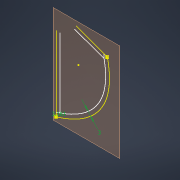
# Autodesk Inventor part: clamsheel sheet surface
Saved by Autodesk Inventor 2021 (Build 250183000, 183)
## iProperties
Created: 2021-02-13
Part Number: clamsheel sheet surface
Material: ABS Plastic
Document SubType Name: Modeling
Designer: vikki
Mass: 19.433 g
Surface Area: 131.842 cm^2
Volume: 18.333 cm^3
Density: 1.06 g/cm^3
Appearance: Brass - Satin
Author: vikki
Autodesk Inventor part; units mm, degrees
ref_plane "YZ Plane" through (0, 0, 0) normal (1, 0, 0) x (0, 1, 0)
ref_plane "XZ Plane" through (0, 0, 0) normal (0, 1, 0) x (-1, 0, 0)
ref_plane "XY Plane" through (0, 0, 0) normal (0, 0, 1) x (1, 0, 0)
ref_plane "Work Plane1" through (0, 0, 0) normal (0, 0, 1) x (1, 0, 0)
sketch "Sketch1" plane through (0, 0, 0) normal (0, 0, 1) x (1, 0, 0)
  spline S0 degree 3 poles (-17.5035, -43.75) (9.5564, -35.6427) (30.0035, -17.8707) (22.4965, 16.6912) knots 1 1 1 1 2 2 2 2 projected
  line L0 (22.4965, 16.6912) -> (-1.9986, 25.6067) projected
  line L1 (-17.5035, 14.75) -> (-17.5035, -43.75) projected
  line L2 (-3.0246, 22.7876) -> (19.8959, 14.4452)
  line L3 (-14.5035, -39.6343) -> (-14.5035, 14.75)
  line L4 (19.8959, 14.4452) -> (19.8959, 17.6377)
  line L5 (-14.5035, -39.6343) -> (-17.5035, -40.6309)
  spline S1 degree 5 poles (19.896, 14.4452) (20.6656, 10.4799) (21.1568, 6.4613) (21.3154, 2.402) (20.7956, -5.2165) (18.5576, -12.5026) (17.0978, -15.7703) (13.3907, -21.8782) (8.4101, -27.002) (5.6606, -29.2971) (0.173, -33.1415) (-5.7852, -36.2005) (-8.6407, -37.4765) (-11.551, -38.6165) (-14.5035, -39.6343) knots 0 0 0 0 0 0 0.283225 0.283225 0.283225 0.531381 0.531381 0.531381 0.781029 0.781029 0.781029 1 1 1 1 1 1
  point P0 (0, 0)
  dimension "d0" = 3
  dimension "d1" = 3.1612
  constraints: 8 end point, 2 parallel, 2 point on line, 1 vertical, 3 other
  measures "d1" distance of L3.start L5.end
extrude "Extrusion1" add sketch "Sketch1" along normal blind 77
body "Solid1"
